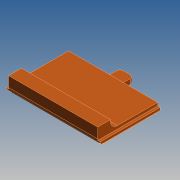
# Autodesk Inventor part: A3_BatteriesTray
Saved by Autodesk Inventor 2020.2 (Build 242310000, 310)
## iProperties
Created: 2021-08-29
Part Number: A3_BatteriesTray
Material: Plastique ABS
Document SubType Name: Modeling
Designer: Samy Francelet
Density: 1.06 g/cm^3
Appearance: Lisse - Orange clair
Author: Samy Francelet
Autodesk Inventor part; units mm, degrees
ref_plane "YZ Plane" through (0, 0, 0) normal (1, 0, 0) x (0, 1, 0)
ref_plane "XZ Plane" through (0, 0, 0) normal (0, 1, 0) x (-1, 0, 0)
ref_plane "XY Plane" through (0, 0, 0) normal (0, 0, 1) x (1, 0, 0)
sketch "Esquisse2" plane through (0, 0, 0) normal (0, 0, 1) x (1, 0, 0)
  line L0 (-26, -17.5) -> (26, -17.5)
  line L1 (26, -17.5) -> (26, 17.5)
  line L2 (26, 17.5) -> (-26, 17.5)
  line L3 (-26, 17.5) -> (-26, -17.5)
  line L4 (-26, -17.5) -> (26, 17.5) construction
  line L5 (26, -17.5) -> (-26, 17.5) construction
  point P0 (0, 0)
  dimension "d0" = 52
  dimension "d1" = 35
  constraints: 12 end point, 2 midpoint, 2 parallel, 1 horizontal, 1 perpendicular
  measures "d0" distance of L2.end L1.end
  measures "d1" distance of L1.end L0.end
extrude "Extrusion1" add sketch "Esquisse2" along normal blind 5
sketch "Esquisse3" plane through (26, -17.5, 0) normal (1, 0, 0) x (0, 0, -1)
  line L0 (0, 0) -> (0, 35) construction
  line L1 (0, 35) -> (-5, 35) construction
  line L2 (-5, 0) -> (-5, 35) construction
  line L3 (0, 0) -> (-5, 0) construction
  line L4 (0, 17.5) -> (-2.5, 17.5) construction
  line L5 (-1.75, 0) -> (-3.25, 0)
  line L6 (-3.25, 0) -> (-3.25, 35)
  line L7 (-3.25, 35) -> (-1.75, 35)
  line L8 (-1.75, 35) -> (-1.75, 0)
  line L9 (-1.75, 0) -> (-3.25, 35) construction
  line L10 (-3.25, 0) -> (-1.75, 35) construction
  dimension "d4" = 2.5
  dimension "d5" = 1.5
  constraints: 14 end point, 2 horizontal, 2 midpoint, 2 parallel, 1 perpendicular, 1 point on line
  measures "d4" distance of L4.start L4.end
  measures "d5" distance of L6.end L7.end
extrude "Extrusion2" add sketch "Esquisse3" along normal blind 1.5
mirror "Symétrie1" about plane through (0, 0, 0) normal (1, 0, 0) of "Extrusion2"
sketch "Esquisse4" plane through (0, 0, 5) normal (0, 0, 1) x (1, 0, 0)
  line L0 (-26, 17.5) -> (-26, -17.5) construction
  line L1 (-26, -17.5) -> (26, -17.5) construction
  line L2 (26, -17.5) -> (26, 17.5) construction
  line L3 (26, 17.5) -> (-26, 17.5) construction
  line L4 (-26, -17.5) -> (26, -17.5)
  line L5 (26, -17.5) -> (26, -10)
  line L6 (26, -10) -> (-26, -10)
  line L7 (-26, -10) -> (-26, -17.5)
  point P0 (0, 0)
  dimension "d8" = 7.5
  constraints: 8 end point, 2 parallel, 1 horizontal, 1 perpendicular, 1 point on line
  measures "d8" distance of L5.end L4.end
extrude "Extrusion3" add sketch "Esquisse4" along normal blind 5
sketch "Esquisse5" plane through (-26, 17.5, 0) normal (0, 1, 0) x (1, 0, 0)
  line L0 (52, 0) -> (0, 0) construction
  line L1 (0, 0) -> (0, -1.75) construction
  line L2 (0, -1.75) -> (-1.5, -1.75) construction
  line L3 (-1.5, -1.75) -> (-1.5, -3.25) construction
  line L4 (0, -3.25) -> (-1.5, -3.25) construction
  line L5 (0, -3.25) -> (0, -5) construction
  line L6 (52, -5) -> (0, -5) construction
  line L7 (52, -3.25) -> (52, -5) construction
  line L8 (52, -3.25) -> (53.5, -3.25) construction
  line L9 (53.5, -1.75) -> (53.5, -3.25) construction
  line L10 (52, -1.75) -> (53.5, -1.75) construction
  line L11 (52, 0) -> (52, -1.75) construction
  line L12 (26, 2) -> (26, -12) construction
  line L13 (-12.5, 0) -> (64.5, 0) construction
  line L14 (26, 0) -> (30, 0) construction
  line L15 (30, 0) -> (22, 0)
  line L16 (22, 0) -> (22, -3)
  line L17 (22, -3) -> (30, -3)
  line L18 (30, -3) -> (30, 0)
  dimension "d11" = 4
  dimension "d12" = 8
  dimension "d13" = 3
  constraints: 10 end point, 2 parallel, 1 horizontal, 1 perpendicular, 1 point on line
  measures "d11" distance of L14.start L14.end
  measures "d12" distance of L17.end L16.end
  measures "d13" distance of L16.end L15.end
extrude "Extrusion4" add sketch "Esquisse5" along normal blind 8
fillet "Congé1" radius 2 2 edges at (4, 25.5, 1.5) (-4, 25.5, 1.5)
fillet "Congé1" radius 4 2 edges at (0, -17.5, 0) (0, -10, 5)
